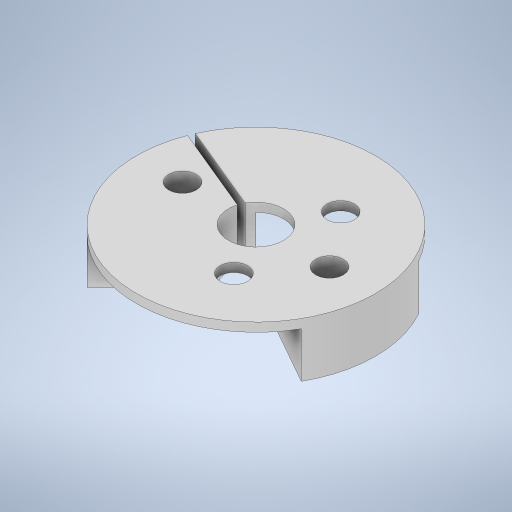
# Autodesk Inventor part: tab4
Saved by Autodesk Inventor 2024 (Build 280153000, 153)
## iProperties
Created: 2023-04-29
Part Number: tab4
Material: Generic
Document SubType Name: Modeling
Designer: Fujitsu
Density: 1 g/cm^3
Appearance: Default
Author: Fujitsu
Autodesk Inventor part; units mm, degrees
ref_plane "YZ Plane" through (0, 0, 0) normal (1, 0, 0) x (0, 1, 0)
ref_plane "XZ Plane" through (0, 0, 0) normal (0, 1, 0) x (-1, 0, 0)
ref_plane "XY Plane" through (0, 0, 0) normal (0, 0, 1) x (1, 0, 0)
sketch "Sketch1" plane through (0, 0, 0) normal (0, 1, 0) x (-1, 0, 0)
  circle A0 centre (0, 0) radius 3.81
  circle A1 centre (0, 0) radius 16.51
  line L0 (-7.4994, -5) -> (-1.1494, -5)
  line L1 (-1.1494, -5) -> (-1.1494, -11.35)
  line L2 (-1.1494, -11.35) -> (-7.4994, -11.35)
  line L3 (-7.4994, -11.35) -> (-7.4994, -5)
  line L4 (-7.4994, 5) -> (-1.1494, 5)
  line L5 (-1.1494, 5) -> (-1.1494, 11.35)
  line L6 (-1.1494, 11.35) -> (-7.4994, 11.35)
  line L7 (-7.4994, 11.35) -> (-7.4994, 5)
  circle A2 centre (-4.3244, -7.3812) radius 1.7526
  circle A3 centre (-4.3244, 7.3812) radius 1.7526
  line L8 (0, 0) -> (-10.16, 0)
  line L9 (0, 0) -> (10.16, 0)
  circle A4 centre (-10.16, 0) radius 1.7526
  circle A5 centre (10.16, 0) radius 1.7526
  line L10 (-4.3244, -8.175) -> (-10.16, 0)
  line L11 (-10.16, 0) -> (-4.3244, 8.175)
  line L12 (0, 0) -> (-7.2422, 4.0875)
  line L13 (0, 0) -> (-7.2422, -4.0875)
  line L14 (-7.2422, -4.0875) -> (-14.378, -8.115)
  line L15 (-7.2422, 4.0875) -> (-14.378, 8.115)
  line L16 (0, 0) -> (11.6743, -11.6743)
  line L17 (0, 0) -> (16.51, 0) construction
  line L18 (0, 0) -> (11.6743, 11.6743)
  line L19 (0, 0) -> (16.51, 0) construction
  line L20 (0, 0) -> (16.51, -6.8387)
  line L21 (0, 0) -> (17.8703, 0) construction
  line L22 (1.062, 0) -> (16.6655, -6.4632)
  line L23 (0.7509, -0.7509) -> (16.3545, -7.2141)
  point P0 (-3.318, 1.8727)
  point P1 (2.6941, 2.6941)
  point P2 (2.6941, -2.6941)
  point P3 (-3.318, -1.8727)
  point P4 (3.3444, -1.8252)
  point P5 (15.0931, -6.6917)
  point P6 (15.4042, -5.9407)
  point P7 (3.6554, -1.0742)
  dimension "d0" = 7.62
  dimension "d1" = 33.02
  dimension "d2" = 6.35
  dimension "d3" = 6.35
  dimension "d4" = 6.35
  dimension "d5" = 6.35
  dimension "d6" = 3.5052
  dimension "d7" = 3.5052
  dimension "d8" = 10.16
  dimension "d9" = 10.16
  dimension "d10" = 3.5052
  dimension "d11" = 3.5052
  dimension "d12" = 45
  dimension "d13" = 45
  dimension "d25" = 22.5
  dimension "d26" = 0.4064
  dimension "d27" = 0.4064
  constraints: 48 end point, 7 horizontal, 6 centre point, 6 parallel, 4 point on circle, 3 equal length, 2 coincident, 2 midpoint, 2 perpendicular, 2 point on line
  measures "d0" diameter of A0
  measures "d1" diameter of A1
  measures "d2" distance of L1.end L2.end
  measures "d3" distance of L0.end L1.end
  measures "d4" distance of L6.end L5.end
  measures "d5" distance of L5.end L4.end
  measures "d6" diameter of A2
  measures "d7" diameter of A3
  measures "d8" distance of L8.start L8.end
  measures "d9" distance of L8.start L9.end
  measures "d10" diameter of A4
  measures "d11" diameter of A5
  measures "d12" angle of L16 L17
  measures "d13" angle of L19 L18
  measures "d25" angle of L20 L21
  measures "d26" distance between parallel lines of L20 L22
  measures "d27" distance between parallel lines of L20 L23
extrude "Extrusion1" add sketch "Sketch1" along normal blind 7.5184 contours A0 L18 A1 L22 | A5 | A3 | L4 L7 L6 L5 | A0 L12 L15 A1 L18 | L22 A1 L20 A0 | A0 L8 A4 L11 L12 | L20 A1 L23 A0 | A0 L13 L10 A4 L8 | L11 A4 L10 L14 A1 L15 | A2 | L0 L1 L2 L3 | A0 L16 A1 L14 L13 | L23 A1 L16 A0 | A4 L10 L8 | L8 L11 A4 | L11 L10 A4
extrude "Extrusion2" cut sketch "Sketch1" along normal blind 6.2992 contours A3 | L4 L7 L6 L5 | A0 L12 L15 A1 L18 | A2 | L0 L1 L2 L3 | A0 L16 A1 L14 L13
hole "Hole1" at (-10.16, 0, 0) at (10.16, 0, 0) at (4.3244, 0, -7.3812) at (4.3244, 0, 7.3812) direction (0, 1, 0) diameter 3.81 end through all clearance for "Flat Head Machine Screw (82)" size "#6" standard "Ansi Unified Screw Threads"
extrude "Extrusion3" cut sketch "Sketch1" along normal blind 7.5184 contours L22 A1 L20 A0 | L20 A1 L23 A0
body "Solid1"
